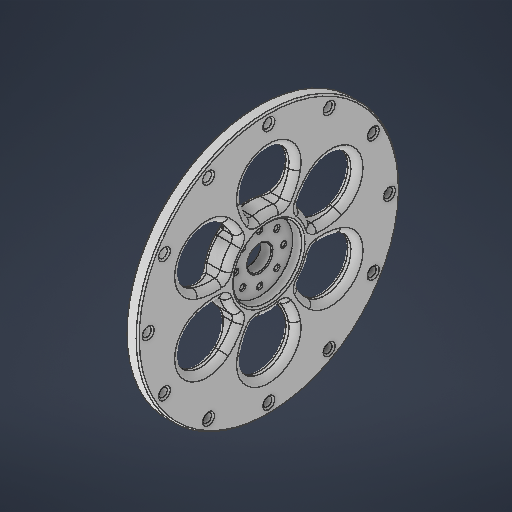
# Autodesk Inventor part: Колесо
Saved by Autodesk Inventor 2025 (Build 290162010, 162A)
## iProperties
Created: 2024-06-21
Part Number: Колесо
Material: Типовые
Document SubType Name: Modeling
Designer: Edward_Higgins
Density: 1 g/cm^3
Appearance: По умолчанию
Author: Edward_Higgins
Autodesk Inventor part; units mm, degrees
ref_plane "YZ Plane" through (0, 0, 0) normal (1, 0, 0) x (0, 1, 0)
ref_plane "XZ Plane" through (0, 0, 0) normal (0, 1, 0) x (-1, 0, 0)
ref_plane "XY Plane" through (0, 0, 0) normal (0, 0, 1) x (1, 0, 0)
sketch "Эскиз1" plane through (0, 0, 0) normal (0, 0, 1) x (1, 0, 0)
  line L0 (0, 0) -> (-61.3454, 0) construction
  line L1 (-14.2142, 60) -> (14.2142, 60) construction
  arc A0 (10, 56.9666) -> (-10, 56.9666) centre (0, 42) ccw
  arc A1 (10.0756, 42.051) -> (10, 56.9666) centre (5, 49.4833) ccw
  arc A2 (-10, 56.9666) -> (-13.9741, 50.1651) centre (-5, 49.4833) ccw
  line L2 (-3, 0) -> (-3, 9.8)
  line L3 (-3, 9.8) -> (-4.5, 9.8)
  line L4 (-4.5, 9.8) -> (-4.5, 12.1237)
  arc A3 (-3.9335, 13.5184) -> (0, 23.2016) centre (-13.8858, 23.2016) ccw
  line L5 (4, 0) -> (4, 15)
  line L6 (-3, 4.05) -> (0, 4.05)
  line L7 (0, 4.05) -> (0, 0)
  arc A4 (-3.9335, 13.5184) -> (-4.5, 12.1237) centre (-2.5, 12.1237) ccw
  line L8 (4, 0) -> (-3, 0)
  line L9 (0, 4.05) -> (4, 4.05)
  arc A5 (-13.9741, 50.1651) -> (-9.9243, 46.5578) centre (-10.5729, 49.9067) ccw
  arc A6 (-1.0482, 43.3008) -> (-9.9243, 46.5578) centre (-8.1847, 37.5756) ccw
  line L10 (4, 15) -> (4, 43.5)
  line L11 (0, 23.2016) -> (0, 43.5)
  line L12 (0, 43.5) -> (4, 43.5)
  point P0 (0, 60)
  point P1 (-4.5, 12.9683)
  point P2 (0, 0)
  dimension "d1" = 120
  dimension "d4" = 19.6
  dimension "d18" = 8.1
  dimension "d19" = 1.5
  dimension "d20" = 3
  dimension "d21" = 18
  dimension "d22" = 7
  dimension "d24" = 9
  dimension "d26" = 2
  dimension "d27" = 3
  dimension "d46" = 10
  dimension "d47" = 30
  dimension "d67" = 4
  dimension "d68" = 87
  constraints: 26 end point, 16 point on circle, 8 tangent, 7 centre point, 6 perpendicular, 4 point on line, 3 horizontal, 3 vertical, 1 equal radius, 1 horizontal alignment, 1 midpoint, 1 vertical alignment
  measures "d1" diameter of L1 L0
  measures "d4" diameter of L3 L0
  measures "d18" diameter of L6 L0
  measures "d19" distance between parallel lines of L2 L4
  measures "d20" distance between parallel lines of L2 L7
  measures "d21" radius of A0
  measures "d22" distance between parallel lines of L5 L2
  measures "d24" radius of A1
  measures "d26" radius of A4
  measures "d27" distance from line of L0.start L2
  measures "d46" distance of A1.centre A2.centre
  measures "d47" diameter of L5.end L0
  measures "d67" distance between parallel lines of L11 L10
  measures "d68" diameter of L12 L0
revolve "Вращение1" add sketch "Эскиз1" angle 360 about axis through (0, 0, 0) along (-1, 0, 0) contours L2 L3 L4 A4 A3 L11 L12 L10 L5 L9 L6
sketch "Эскиз4" plane through (-3, 0, 0) normal (-1, 0, 0) x (0, 0, 1)
  circle A0 centre (-8, 0) radius 0.75
  circle A1 centre (0, 0) radius 8 construction
  dimension "d30" = 16
  dimension "d31" = 1.5
  constraints: 2 horizontal alignment, 1 centre point, 1 coincident, 2 other
  measures "d31" diameter of A0
extrude "Выдавливание2" cut sketch "Эскиз4" against normal through all
pattern_circular "Круговой массив3" count 8 over 360 about axis through (-3.75, 0, 0) along (-1, 0, 0) of "Выдавливание2"
sketch "Эскиз6" plane through (4, 0, 0) normal (1, 0, 0) x (0, 0, -1)
  circle A0 centre (0, 0) radius 11.5
  dimension "d37" = 23
  constraints: 1 centre point, 1 coincident
  measures "d37" diameter of A0
extrude "Выдавливание3" cut sketch "Эскиз6" against normal blind 3 draft -10
chamfer "Фаска1" distance 0.3 angle 45 19 edges at (1, -4.05, 0) (-3, -4.05, 0) (-4.5, -9.8, 0) (1, -8.75, 0) (1, -6.1872, -6.1872) (1, 0, -8.75) (1, 6.1872, -6.1872) (1, 8.75, 0) (1, 6.1872, 6.1872) (1, 0, 8.75) (1, -6.1872, 6.1872) (-3, -6.1872, 6.1872) (-3, -8.75, 0) (-3, -6.1872, -6.1872) (-3, 0, -8.75) (-3, 6.1872, -6.1872) (-3, 8.75, 0) (-3, 6.1872, 6.1872) (-3, 0, 8.75)
sketch "Эскиз8" plane through (4, 0, 0) normal (1, 0, 0) x (0, 0, -1)
  arc A0 (8.5388, 21.9792) -> (-8.5388, 21.9792) centre (0, 23.7119) ccw
  arc A1 (3.4958, 14.3304) -> (-3.4958, 14.3304) centre (0, 0) ccw
  arc A2 (5.6118, 15.1315) -> (8.5388, 21.9792) centre (-9.4973, 25.6392) ccw
  arc A3 (-8.5388, 21.9792) -> (-5.6118, 15.1315) centre (9.4973, 25.6392) ccw
  arc A4 (-5.6118, 15.1315) -> (-3.4958, 14.3304) centre (-3.9698, 16.2734) ccw
  arc A5 (3.4958, 14.3304) -> (5.6118, 15.1315) centre (3.9698, 16.2734) ccw
  dimension "d69" = 2
  constraints: 12 point on circle, 6 centre point, 6 tangent, 2 horizontal alignment, 1 coincident, 1 equal radius, 1 vertical alignment
  measures "d69" radius of A4
extrude "Выдавливание4" cut sketch "Эскиз8" against normal blind 15
fillet "Сопряжение5" radius 2 6 edges at (4, 32.4248, 0) (4, 18.4058, -7.4253) (4, 14.403, -4.678) (4, 14.7507, 0) (4, 14.403, 4.678) (4, 18.4058, 7.4253)
fillet "Сопряжение5" radius 1 9 edges at (0, 21.7918, -8.4997) (0, 32.4248, 0) (0, 21.7918, 8.4997) (-0.5242, 18.0169, 7.2537) (-2.5407, 14.4329, 4.7524) (-2.8678, 14.6452, -1.7605) (-2.8678, 14.6452, 1.7605) (-2.5404, 14.4331, -4.7529) (-0.5242, 18.0169, -7.2537)
pattern_circular "Круговой массив5" count 6 over 360 about axis through (0.5, 0, 0) along (-1, 0, 0) of "Сопряжение5", "Выдавливание4"
sketch "Эскиз9" plane through (4, 0, 0) normal (1, 0, 0) x (0, 0, -1)
  circle A0 centre (0, 40) radius 1.5
  point P0 (0, 0)
  dimension "d77" = 3
  dimension "d78" = 40
  constraints: 1 centre point, 1 vertical alignment
  measures "d77" diameter of A0
  measures "d78" distance of point (0, 0) A0.centre
extrude "Выдавливание5" cut sketch "Эскиз9" against normal up to surface (4 mm away)
chamfer "Фаска4" distance 0.5 angle 45 2 edges at (4, 40, 1.5) (0, 40, 1.5)
pattern_circular "Круговой массив6" count 12 over 360 about axis through (2, 0, 0) along (-1, 0, 0) of "Выдавливание5", "Фаска4"
chamfer "Фаска3" distance 0.5 angle 45 3 edges at (0, -43.5, 0) (4, -43.5, 0) (4, 0, 11.5)
